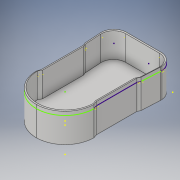
# Autodesk Inventor part: Random Object
Saved by Autodesk Inventor 2018 (Build 220112000, 112)
## iProperties
Created: 2019-03-26
Part Number: Random Object
Material: Generic
Document SubType Name: Modeling
Designer: This kid
Density: 1 g/cm^3
Appearance: Default
Author: This kid
Autodesk Inventor part; units mm, degrees
ref_plane "YZ Plane" through (0, 0, 0) normal (1, 0, 0) x (0, 1, 0)
ref_plane "XZ Plane" through (0, 0, 0) normal (0, 1, 0) x (-1, 0, 0)
ref_plane "XY Plane" through (0, 0, 0) normal (0, 0, 1) x (1, 0, 0)
sketch "Sketch1" plane through (0, 0, 0) normal (0, 0, 1) x (1, 0, 0)
  point P0 (0, 0)
sketch "Sketch2" plane through (0, 0, 0) normal (0, 1, 0) x (-1, 0, 0)
  line L0 (29.4419, 0) -> (29.4988, 0)
  arc A0 (58.9407, -29.4419) -> (29.4988, 0) centre (29.4988, -29.4419) ccw
  arc A1 (29.4419, 0) -> (0, -29.4419) centre (29.4419, -29.4419) ccw
  line L1 (0, -29.4419) -> (1.3334, -33.4091)
  line L2 (1.3334, -33.4091) -> (1.3334, -74.6587)
  line L3 (1.3334, -74.6587) -> (0, -77.6285)
  line L4 (0, -77.6285) -> (-1.0327, -97.9222)
  line L5 (58.9407, -29.4419) -> (57.7766, -33.4091)
  line L6 (57.7766, -33.4091) -> (57.7766, -76.7951)
  line L7 (57.7766, -76.7951) -> (58.9407, -78.9752)
  line L8 (58.9407, -78.9752) -> (59.9743, -95.7523)
  line L9 (59.9743, -95.7523) -> (60.0189, -96.4757)
  line L10 (-1.0327, -97.9222) -> (-0.9556, -96.5463)
  line L11 (11.7245, -109.9566) -> (47.3429, -109.9566)
  arc A2 (47.3429, -109.9566) -> (60.0189, -96.4757) centre (47.3429, -97.2566) ccw
  arc A3 (-0.9556, -96.5463) -> (11.7245, -109.9566) centre (11.7245, -97.2566) ccw
  point P0 (0, 0)
  point P1 (58.9407, 0)
  dimension "d5" = 29.4419
  dimension "d6" = 41.2496
  dimension "d7" = 20.32
  dimension "d8" = 12.7
  constraints: 24 end point, 8 point on circle, 6 tangent, 4 centre point, 3 vertical, 2 equal radius, 2 horizontal, 2 point on line, 3 other
  measures "d5" radius of A0
  measures "d6" distance of L1.end L2.end
  measures "d7" distance of L3.end L4.end
  measures "d8" radius of A2
extrude "Extrusion1" add sketch "Sketch2" along normal blind 29.5148
sketch "Sketch3" plane through (0, 29.5148, 0) normal (0, 1, 0) x (1, 0, 0)
  line L0 (-29.7463, 1.6533) -> (-29.8195, 1.6533)
  arc A0 (-58.3691, 30.2029) -> (-29.8195, 1.6533) centre (-29.8195, 30.2029) ccw
  arc A1 (-29.7463, 1.6533) -> (-1.1967, 30.2029) centre (-29.7463, 30.2029) ccw
  line L1 (-1.1967, 30.2029) -> (-2.4901, 33.4321)
  line L2 (-2.4901, 33.4321) -> (-2.4901, 73.4442)
  line L3 (-2.4901, 73.4442) -> (-0.5766, 76.9439)
  line L4 (-0.5766, 76.9439) -> (0.4251, 96.6289)
  line L5 (-58.3691, 30.2029) -> (-56.62, 33.4321)
  line L6 (-56.62, 33.4321) -> (-56.62, 75.5165)
  line L7 (-56.62, 75.5165) -> (-57.7491, 78.2503)
  line L8 (-57.7491, 78.2503) -> (-58.7517, 94.5241)
  line L9 (-58.7517, 94.5241) -> (-58.7949, 95.2257)
  line L10 (0.4251, 96.6289) -> (0.3503, 95.2942)
  line L11 (-11.9494, 108.3022) -> (-46.4992, 108.3022)
  arc A2 (-46.4992, 108.3022) -> (-58.7949, 95.2257) centre (-46.4992, 95.9832) ccw
  arc A3 (0.3503, 95.2942) -> (-11.9494, 108.3022) centre (-11.9494, 95.9832) ccw
  line L12 (-2.4901, 52.1447) -> (-2.4901, 53.4382) construction
  line L13 (-57.7766, 76.7951) -> (-57.7766, 33.4091) construction
  line L14 (-57.7766, 54.1324) -> (-56.62, 54.1324) construction
  arc A4 (-58.9407, 29.4419) -> (-29.4988, 0) centre (-29.4988, 29.4419) ccw construction
  line L15 (-29.4988, 0) -> (-29.4988, 1.6544) construction
  line L16 (-28.1015, 108.3022) -> (-28.1015, 109.9566) construction
  line L17 (-11.7245, 109.9566) -> (-47.3429, 109.9566) construction
  line L18 (-2.4901, 53.4382) -> (-1.3334, 53.4382) construction
  line L19 (-1.3334, 33.4091) -> (-1.3334, 74.6587) construction
  point P0 (0, 0)
  point P1 (-1.2057, 1.6533)
  point P2 (-58.3782, 1.6533)
  dimension "d9" = 28.5496
  dimension "d10" = 40.0121
  dimension "d11" = 19.7104
  dimension "d12" = 12.319
  constraints: 34 end point, 9 point on circle, 7 point on line, 6 tangent, 4 centre point, 3 parallel, 2 equal radius, 2 perpendicular, 1 horizontal, 1 midpoint, 1 vertical
  measures "d9" radius of A0
  measures "d10" distance of L1.end L2.end
  measures "d11" distance of L3.end L4.end
  measures "d12" radius of A2
extrude "Extrusion2" cut sketch "Sketch3" against normal blind 25.4
sketch "Sketch4" plane through (0, 29.5148, 0) normal (0, 1, 0) x (1, 0, 0)
  point P0 (0, 0)
sketch "Sketch5" plane through (-11.7245, 0, -109.9566) normal (0, 0, -1) x (-1, 0, 0)
  line L0 (35.6184, 26.9603) -> (35.6184, 25.922)
  line L1 (35.6184, 0) -> (35.6184, 29.5148) projected
  line L2 (0, 0) -> (0, 29.5148) projected
  point P0 (-11.7245, 0)
  constraints: 2 end point, 1 point on line
sketch3d "3D Sketch1"
sketch "Sketch6" plane through (0, 29.5148, 0) normal (0, 1, 0) x (1, 0, 0)
  point P0 (0, 0)
ref_plane "Work Plane3" through (-47.3429, 25.922, -109.9566) normal (0, 1, 0) x (1, 0, 0)
sketch "Sketch7" plane through (-47.3429, 25.922, -109.9566) normal (0, 1, 0) x (1, 0, 0)
  line L0 (46.0094, -76.5475) -> (46.0094, -35.2979)
  line L1 (46.0094, -35.2979) -> (47.3429, -32.3281)
  line L2 (47.3429, -32.3281) -> (48.2985, -13.4103)
  line L3 (48.2985, -13.4103) -> (48.3756, -12.0344)
  line L4 (46.0094, -76.5475) -> (47.3429, -80.5147)
  line L5 (0, 0) -> (35.6184, 0)
  line L6 (-12.676, -13.4809) -> (-11.5978, -30.9814)
  line L7 (-11.5978, -30.9814) -> (-10.4337, -33.1615)
  line L8 (-10.4337, -33.1615) -> (-10.4337, -76.5475)
  line L9 (-10.4337, -76.5475) -> (-11.5978, -80.5147)
  arc A0 (-11.5978, -80.5147) -> (47.3429, -80.5147) centre (17.8725, -80.5147) ccw
  arc A1 (48.3756, -12.0344) -> (35.6184, 0) centre (35.6184, -12.7789) ccw
  line L10 (-12.676, -13.4809) -> (-11.5978, -30.9814) projected
  arc A2 (0, 0) -> (-12.676, -13.4809) centre (0, -12.7) ccw
  point P0 (47.3429, -109.9566)
  constraints: 20 end point, 6 point on circle, 3 centre point, 2 tangent, 2 vertical, 1 horizontal
body "Solid1"
